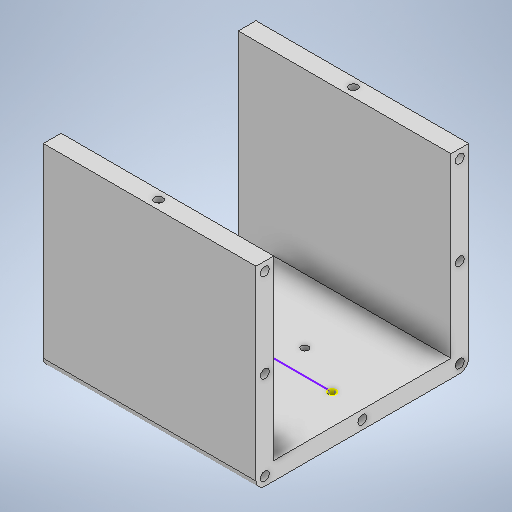
# Autodesk Inventor part: Fuselage_Body_Piece
Saved by Autodesk Inventor 2025.1 (Build 291241020, 241B)
## iProperties
Created: 2025-02-15
Part Number: Fuselage_Body_Piece
Material: Generic
Document SubType Name: Modeling
Designer: smyth
Density: 1 g/cm^3
Appearance: Default
Author: smyth
Autodesk Inventor part; units mm, degrees
ref_plane "YZ Plane" through (0, 0, 0) normal (1, 0, 0) x (0, 1, 0)
ref_plane "XZ Plane" through (0, 0, 0) normal (0, 1, 0) x (-1, 0, 0)
ref_plane "XY Plane" through (0, 0, 0) normal (0, 0, 1) x (1, 0, 0)
sketch "Sketch1" plane through (0, 0, 0) normal (0, 1, 0) x (-1, 0, 0)
  point P0 (0, 0)
sketch "Sketch2" plane through (0, 0, 0) normal (0, 1, 0) x (-1, 0, 0)
  line L0 (-76.2, 76.2) -> (76.2, 76.2)
  line L1 (76.2, 76.2) -> (76.2, -76.2)
  line L2 (76.2, -76.2) -> (-76.2, -76.2)
  line L3 (-76.2, -76.2) -> (-76.2, 76.2)
  line L4 (-76.2, 76.2) -> (76.2, -76.2) construction
  line L5 (76.2, 76.2) -> (-76.2, -76.2) construction
  point P0 (0, 0)
  dimension "d0" = 152.4
  dimension "d1" = 152.4
  constraints: 12 end point, 2 midpoint, 2 parallel, 1 horizontal, 1 perpendicular
  measures "d0" distance of L1.end L2.end
  measures "d1" distance of L0.end L1.end
extrude "Extrusion1" add sketch "Sketch2" along normal blind 12.7
sketch "Sketch3" plane through (0, 12.7, 0) normal (0, 1, 0) x (1, 0, 0)
  line L0 (76.2, 76.2) -> (-76.2, 76.2) projected
  line L1 (76.2, -76.2) -> (76.2, 76.2) projected
  line L2 (-76.2, 76.2) -> (76.2, 76.2)
  line L3 (76.2, 76.2) -> (76.2, 63.5)
  line L4 (76.2, 63.5) -> (-76.2, 63.5)
  line L5 (-76.2, 63.5) -> (-76.2, 76.2)
  line L6 (-76.2, -76.2) -> (76.2, -76.2)
  line L7 (76.2, -76.2) -> (76.2, -63.5)
  line L8 (76.2, -63.5) -> (-76.2, -63.5)
  line L9 (-76.2, -63.5) -> (-76.2, -76.2)
  point P0 (0, 0)
  point P1 (76.2, -76.2)
  dimension "d4" = 12.7
  dimension "d5" = 12.7
  dimension "d15" = 152.4
  constraints: 16 end point, 4 parallel, 2 horizontal, 2 perpendicular, 2 point on line
  measures "d4" distance between parallel lines of L4 L0
  measures "d5" distance between parallel lines of L8 L6
  measures "d15" distance of L6.start L6.end
extrude "Extrusion2" add sketch "Sketch3" along normal blind 127
fillet "Fillet1" radius 6.35 2 edges at (0, 0, 76.2) (0, 0, -76.2)
sketch "Sketch4" plane through (76.2, 12.7, -63.5) normal (1, 0, 0) x (0, 0, -1)
  circle A0 centre (-133.35, 120.65) radius 3.175
  circle A1 centre (-133.35, -6.35) radius 3.175
  circle A2 centre (-133.35, 57.15) radius 3.175
  circle A3 centre (6.35, 120.65) radius 3.175
  circle A4 centre (6.35, -6.35) radius 3.175
  circle A5 centre (6.35, 57.15) radius 3.175
  circle A6 centre (-63.5, -6.35) radius 3.175
  point P0 (-63.5, -12.7)
  dimension "d9" = 127
  constraints: 7 centre point
  measures "d9" distance of A1.centre A0.centre
extrude "Extrusion3" cut sketch "Sketch4" against normal blind 12.7
sketch "Sketch5" plane through (-76.2, 12.7, 63.5) normal (-1, 0, 0) x (0, 0, 1)
  circle A0 centre (-133.35, 120.65) radius 3.175 projected
  circle A1 centre (-133.35, 120.65) radius 3.175
  circle A2 centre (-133.35, 57.15) radius 3.175 projected
  circle A3 centre (-133.35, 57.15) radius 3.175
  circle A4 centre (-133.35, -6.35) radius 3.175 projected
  circle A5 centre (-133.35, -6.35) radius 3.175
  circle A6 centre (-63.5, -6.35) radius 3.175 projected
  circle A7 centre (-63.5, -6.35) radius 3.175
  circle A8 centre (6.35, -6.35) radius 3.175 projected
  circle A9 centre (6.35, -6.35) radius 3.175
  circle A10 centre (6.35, 57.15) radius 3.175 projected
  circle A11 centre (6.35, 57.15) radius 3.175
  circle A12 centre (6.35, 120.65) radius 3.175 projected
  circle A13 centre (6.35, 120.65) radius 3.175
  line L0 (6.35, -12.7) -> (-133.35, -12.7) projected
  point P0 (-63.5, -12.7)
  dimension "d20" = 69.85
  constraints: 7 centre point, 7 coincident
  measures "d20" distance from line of L0 A11.centre
sketch "Sketch6" plane through (0, 139.7, 0) normal (0, 1, 0) x (1, 0, 0)
  line L0 (76.2, 69.85) -> (-76.2, 69.85) projected
  circle A0 centre (0, 69.85) radius 3
  line L1 (-76.2, -69.85) -> (76.2, -69.85) projected
  circle A1 centre (0, -69.85) radius 3
  point P0 (0, 0)
  dimension "d16" = 6
  dimension "d17" = 6
  constraints: 2 centre point, 2 midpoint
  measures "d16" diameter of A0
  measures "d17" diameter of A1
extrude "Extrusion5" cut sketch "Sketch6" against normal blind 4
extrude "Extrusion6" cut sketch "Sketch5" against normal blind 12.7
sketch "Sketch7" plane through (0, 12.7, 0) normal (0, 1, 0) x (1, 0, 0)
  line L0 (76.2, 0) -> (63.5, 0)
  line L1 (63.5, 3.175) -> (63.5, -3.175) projected
  line L2 (63.5, 0) -> (57.15, 0)
  circle A0 centre (54.5465, 0) radius 2.6035
  line L3 (51.943, 0) -> (-35.687, 0)
  line L4 (-35.687, 0) -> (-35.687, 35.56)
  line L5 (-35.687, 35.56) -> (-35.687, -35.56)
  circle A1 centre (-35.687, 38.1635) radius 2.6035
  circle A2 centre (-35.687, -38.1635) radius 2.6035
  point P0 (0, 0)
  dimension "d28" = 5.207
  dimension "d29" = 5.207
  dimension "d23" = 6.35
  dimension "d24" = 5.207
  dimension "d25" = 87.63
  dimension "d26" = 35.56
  dimension "d27" = 71.12
  constraints: 10 end point, 2 horizontal, 2 point on circle, 2 vertical alignment, 1 centre point, 1 midpoint, 1 perpendicular, 1 point on line, 4 other
  measures "d23" distance of L0.end L2.end
  measures "d24" diameter of A0
  measures "d25" distance of L3.start L3.end
  measures "d26" distance of L3.end L4.end
  measures "d27" distance of L4.end L5.end
extrude "Extrusion7" cut sketch "Sketch7" against normal blind 3.9878
sketch "Sketch8" plane through (0, 12.7, 0) normal (0, 1, 0) x (1, 0, 0)
  circle A0 centre (54.5465, 0) radius 2.6035 projected
  line L0 (51.943, 0) -> (-76.2, 0)
  point P0 (0, 0)
  constraints: 2 end point, 1 horizontal, 1 horizontal alignment, 1 other
sketch "Sketch9" plane through (0, 12.7, 0) normal (0, 1, 0) x (1, 0, 0)
  point P0 (0, 0)
sketch "Sketch10" plane through (0, 12.7, 0) normal (0, 1, 0) x (1, 0, 0)
  line L0 (57.15, -63.5) -> (57.15, -52.07)
  line L1 (57.15, -57.785) -> (-19.177, -57.785)
  line L2 (-76.2, -63.5) -> (76.2, -63.5) projected
  line L3 (13.97, -63.5) -> (13.97, -52.07)
  line L4 (11.1125, -52.07) -> (17.4625, -52.07)
  circle A0 centre (14.2875, -49.4665) radius 2.6035
  circle A1 centre (59.7535, -57.785) radius 2.6035
  line L5 (-19.177, -61.9125) -> (-19.177, -53.133)
  circle A2 centre (-21.7805, -57.785) radius 2.6035
  point P0 (0, 0)
  dimension "d32" = 11.43
  dimension "d33" = 76.327
  dimension "d36" = 5.207
  dimension "d37" = 5.207
  dimension "d38" = 5.207
  constraints: 10 end point, 3 centre point, 3 tangent, 3 vertical, 2 horizontal, 1 midpoint, 1 point on line
  measures "d32" distance of L0.start L0.end
  measures "d33" distance of L1.start L1.end
  measures "d36" diameter of A2
  measures "d37" diameter of A0
  measures "d38" diameter of A1
extrude "Extrusion8" cut sketch "Sketch10" against normal blind 3.9878 contours A2 | A0 | A1
sketch "Sketch11" plane through (0, 0, 0) normal (0, -1, 0) x (1, 0, 0)
  line L0 (17.526, -17.526) -> (-17.526, -17.526)
  line L1 (-17.526, -17.526) -> (-17.526, 17.526)
  line L2 (-17.526, 17.526) -> (17.526, 17.526)
  line L3 (17.526, 17.526) -> (17.526, -17.526)
  line L4 (17.526, -17.526) -> (-17.526, 17.526) construction
  line L5 (-17.526, -17.526) -> (17.526, 17.526) construction
  circle A0 centre (-50.8, 55.5625) radius 2.6035
  circle A1 centre (-17.526, 17.526) radius 2.6035
  circle A2 centre (-17.526, -17.526) radius 2.6035
  circle A3 centre (17.526, -17.526) radius 2.6035
  circle A4 centre (17.526, 17.526) radius 2.6035
  point P0 (0, 0)
  dimension "d39" = 35.052
  dimension "d40" = 35.052
  dimension "d41" = 5.207
  dimension "d42" = 5.207
  dimension "d43" = 5.207
  dimension "d44" = 5.207
  dimension "d45" = 5.207
  constraints: 12 end point, 5 centre point, 4 coincident, 2 midpoint, 2 parallel, 1 horizontal, 1 perpendicular
  measures "d39" distance of L1.end L2.end
  measures "d40" distance of L0.end L1.end
  measures "d41" diameter of A0
  measures "d42" diameter of A3
  measures "d43" diameter of A2
  measures "d44" diameter of A1
  measures "d45" diameter of A4
extrude "Extrusion9" cut sketch "Sketch11" along normal blind 25.4 and the other way blind 25.4 contours A2 L1 L0 | L0 L1 A2 | A3 L3 L0 | L0 L3 A3 | A1 L2 L1 | L1 L2 A1 | A4 L2 L3 | L3 L2 A4
sketch "Sketch13" plane through (0, 12.7, 0) normal (0, 1, 0) x (1, 0, 0)
  circle A0 centre (0, 0) radius 2.6035
  dimension "d54" = 5.207
  constraints: 1 centre point, 1 coincident
  measures "d54" diameter of A0
extrude "Extrusion11" cut sketch "Sketch13" against normal blind 25.4
body "Solid1"
